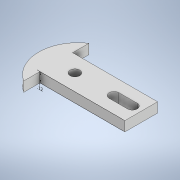
# Autodesk Inventor part: FPV_Motor_Holder
Saved by Autodesk Inventor 2020 (Build 240168000, 168)
## iProperties
Created: 2020-11-25
Part Number: FPV_Motor_Holder
Material: Generic
Document SubType Name: Modeling
Designer: wongz
Density: 1 g/cm^3
Appearance: Default
Author: wongz
Autodesk Inventor part; units mm, degrees
ref_plane "YZ Plane" through (0, 0, 0) normal (1, 0, 0) x (0, 1, 0)
ref_plane "XZ Plane" through (0, 0, 0) normal (0, 1, 0) x (-1, 0, 0)
ref_plane "XY Plane" through (0, 0, 0) normal (0, 0, 1) x (1, 0, 0)
sketch "Sketch1" plane through (0, 0, 0) normal (0, 1, 0) x (-1, 0, 0)
  line L0 (0, 0) -> (-26, 0)
  line L1 (-26, 0) -> (-26, -10)
  line L2 (-26, -10) -> (0, -10)
  line L3 (0, -10) -> (0, 0)
  line L4 (0, 0) -> (0, 5)
  line L5 (0, -10) -> (0, -15)
  circle A0 centre (-5.7, -5) radius 1.5
  arc A1 (-23.3, -3.5) -> (-23.3, -6.5) centre (-23.3, -5) ccw
  line L6 (-23.3, -3.5) -> (-17.6724, -3.5)
  line L7 (-17.6724, -3.5) -> (-17.6724, -6.5)
  line L8 (-17.6724, -6.5) -> (-23.3, -6.5)
  arc A2 (-17.6724, -6.5) -> (-17.6724, -3.5) centre (-17.6724, -5) ccw
  arc A3 (0, -15) -> (0, 5) centre (-6.6332, -5) ccw
  dimension "d0" = 26
  dimension "d1" = 10
  dimension "d5" = 3
  dimension "d7" = 3
  dimension "d8" = 3
  dimension "d9" = 12
  constraints: 18 end point, 6 point on circle, 4 centre point, 3 parallel, 2 horizontal, 2 perpendicular, 2 vertical, 1 midpoint
  measures "d0" distance of L2.end L1.end
  measures "d1" distance of L1.end L0.end
  measures "d5" diameter of A0
  measures "d7" diameter of A1
  measures "d8" diameter of A2
  measures "d9" radius of A3
extrude "Extrusion1" add sketch "Sketch1" along normal blind 3
body "Solid1"
